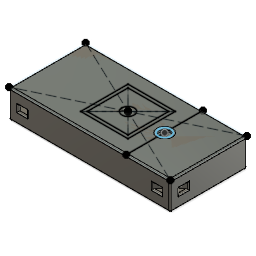
box1 (Autodesk Fusion 360 design; units mm, degrees)
Autodesk Fusion 360 part; units mm, degrees
note: some values were not read from the file. Set by a fixed rule: which sketch regions a step uses.
sketch "Sketch1" plane through (0, 0, 0) normal (0, 1, 0) x (1, 0, 0)
  line L0 (-95, -45) -> (95, -45)
  line L1 (95, -45) -> (95, 45)
  line L2 (95, 45) -> (-95, 45)
  line L3 (-95, 45) -> (-95, -45)
  line L4 (-95, -45) -> (95, 45) construction
  line L5 (95, -45) -> (-95, 45) construction
  line L6 (-99, -49) -> (99, -49)
  line L7 (99, -49) -> (99, 49)
  line L8 (99, 49) -> (-99, 49)
  line L9 (-99, 49) -> (-99, -49)
  line L10 (-99, -49) -> (99, 49) construction
  line L11 (99, -49) -> (-99, 49) construction
  line L12 (-57.3192, 45) -> (-19.6385, 45)
  line L13 (-19.6385, 45) -> (-19.6385, -45)
  line L14 (-19.6385, -45) -> (-57.3192, -45)
  line L15 (-57.3192, -45) -> (-57.3192, 45)
  line L16 (19.6385, 45) -> (57.3192, 45)
  line L17 (57.3192, 45) -> (57.3192, -45)
  line L18 (57.3192, -45) -> (19.6385, -45)
  line L19 (19.6385, -45) -> (19.6385, 45)
  line L20 (-57.3192, -35) -> (-19.6385, -35) construction
  line L21 (19.6385, -35) -> (57.3192, -35) construction
  line L22 (57.3192, -20) -> (95, -20) construction
  line L23 (-95, -29.9905) -> (-57.3192, -29.9905) construction
  line L24 (-87.5, 49) -> (87.5, 49)
  line L25 (-99, -49) -> (99, -49)
  line L26 (99, -49) -> (99, -143)
  line L27 (99, -143) -> (-99, -143)
  line L28 (-99, -143) -> (-99, -49)
  line L29 (-95, -49) -> (95, -49)
  line L30 (95, -49) -> (95, -139)
  line L31 (95, -139) -> (-95, -139)
  line L32 (-95, -139) -> (-95, -49)
  line L33 (-95, -49) -> (-75, -49)
  line L34 (-75, -49) -> (-75, -74)
  line L35 (-75, -74) -> (-95, -74)
  line L36 (-95, -74) -> (-95, -49)
  line L37 (-95, -139) -> (-75, -139)
  line L38 (-75, -139) -> (-75, -119)
  line L39 (-75, -119) -> (-95, -119)
  line L40 (-95, -119) -> (-95, -139)
  line L41 (95, -139) -> (75, -139)
  line L42 (75, -139) -> (75, -119)
  line L43 (75, -119) -> (95, -119)
  line L44 (95, -119) -> (95, -139)
  line L45 (95, -49) -> (75, -49)
  line L46 (75, -49) -> (75, -74)
  line L47 (75, -74) -> (95, -74)
  line L48 (95, -74) -> (95, -49)
  dimension "d1" = 190
  dimension "d2" = 90
  dimension "d4" = 4
  dimension "d5" = 4
  dimension "d26" = 4
  dimension "d27" = 4
  dimension "d28" = 4
  dimension "d29" = 20
  dimension "d30" = 25
  dimension "d31" = 20
  dimension "d32" = 20
  dimension "d33" = 20
  dimension "d34" = 20
  dimension "d35" = 20
  dimension "d36" = 25
  dimension "d48" = 90
  constraint horizontal L0
  constraint perpendicular L0 L1
  constraint parallel L0 L2
  constraint parallel L1 L3
  constraint coincident L4 origin
  constraint coincident L5 origin
  constraint horizontal L6
  constraint perpendicular L6 L7
  constraint parallel L6 L8
  constraint parallel L7 L9
  constraint coincident L10 origin
  constraint coincident L11 origin
  constraint horizontal L12
  constraint vertical L13
  constraint horizontal L14
  constraint vertical L15
  constraint coincident L0 L13.end
  constraint coincident L2 L12.start
  constraint horizontal L16
  constraint vertical L17
  constraint horizontal L18
  constraint vertical L19
  constraint coincident L0 L17.end
  constraint coincident L2 L16.start
  constraint coincident L13 L20.end
  constraint perpendicular L13 L20
  constraint coincident L19 L21.start
  constraint coincident L17 L21.end
  constraint perpendicular L17 L21
  constraint coincident L17 L22.start
  constraint coincident L1 L22.end
  constraint perpendicular L1 L22
  constraint coincident L15 L20.start
  constraint equal L20 L21
  constraint equal L21 L22
  constraint coincident L3 L23.start
  constraint coincident L15 L23.end
  constraint perpendicular L15 L23
  constraint equal L20 L23
  constraint horizontal L24
  constraint coincident L8 L24.start
  constraint horizontal L25
  constraint vertical L26
  constraint horizontal L27
  constraint vertical L28
  constraint collinear L7 L26
  constraint horizontal L29
  constraint vertical L30
  constraint horizontal L31
  constraint vertical L32
  constraint coincident L6 L29.start
  constraint horizontal L33
  constraint vertical L34
  constraint horizontal L35
  constraint vertical L36
  constraint horizontal L37
  constraint vertical L38
  constraint horizontal L39
  constraint vertical L40
  constraint horizontal L41
  constraint vertical L42
  constraint horizontal L43
  constraint vertical L44
  constraint horizontal L45
  constraint vertical L46
  constraint horizontal L47
  constraint vertical L48
  measures "d1" distance of L1.end L2.end
  measures "d2" distance of L0.end L1.end
  measures "d4" distance of L2 L8
  measures "d5" distance of L3 L9
  measures "d26" distance of L26 L30
  measures "d27" distance of L28 L32
  measures "d28" distance of L27 L31
  measures "d29" distance of L29.start L33.end
  measures "d30" distance of L29.start L35.end
  measures "d31" distance of L31.end L37.end
  measures "d32" distance of L31.end L39.end
  measures "d33" distance of L30.end L41.end
  measures "d34" distance of L30.end L43.end
  measures "d35" distance of L29.end L45.end
  measures "d36" distance of L29.end L47.end
  measures "d48" distance of L25 L31
extrude "Extrude1" add sketch "Sketch1" along normal blind 31 from surface at 4 contours L6 L7 L8 L9 L24 L25 L29 L33 L45 makes body 1
extrude "Extrude2" add sketch "Sketch1" along normal blind 4 contours L0 L2 L3 L15 | L0 L2 L12 L13 L14 L15 | L0 L2 L13 L19 | L0 L2 L16 L17 L18 L19 | L0 L1 L2 L17 | L6 L7 L8 L9 L24 L25 L29 L33 L45 bodies 1
sketch "Sketch2" plane through (-99, 0, 0) normal (-1, 0, 0) x (0, 0, 1)
  line L0 (49, 0) -> (49, 35)
  line L1 (49, 35) -> (-49, 35)
  line L2 (-49, 35) -> (-49, 0)
  line L3 (-49, 0) -> (49, 0)
  line L4 (-45, 4) -> (45, 4)
  line L5 (45, 4) -> (45, 31)
  line L6 (45, 31) -> (-45, 31)
  line L7 (-45, 31) -> (-45, 4)
  line L8 (-45, 4) -> (45, 31) construction
  line L9 (45, 4) -> (-45, 31) construction
  line L10 (-49, 35) -> (49, 0) construction
  line L11 (-49, 0) -> (49, 35) construction
  line L12 (-49, 0) -> (49, 0)
  point P0 (0, 17.5)
  point P1 (0, 17.5)
  dimension "d12" = 90
  dimension "d15" = 4
  constraint horizontal L4
  constraint perpendicular L4 L5
  constraint parallel L4 L6
  constraint parallel L5 L7
  constraint coincident L8 P1
  constraint coincident L9 P1
  constraint coincident L1.end L2.start
  constraint coincident L0.start L3.end
  constraint coincident L2.end L3.start
  constraint coincident L0.end L1.start
  constraint midpoint L10 P1
  constraint coincident P1 P0
  measures "d12" distance of L5 L7
  measures "d15" distance of L4 L12
extrude "Extrude3" cut sketch "Sketch2" against normal blind 10 contours L4 L5 L6 L7 bodies 1
sketch "Sketch3" plane through (0, 0, 0) normal (0, 1, 0) x (1, 0, 0)
extrude "Extrude4" cut sketch "Sketch1" along normal blind 20 contours L0 L2 L3 L15 | L0 L2 L13 L19 | L0 L1 L2 L17 bodies 1
sketch "Sketch5" plane through (0, 0, -49) normal (0, 0, -1) x (-1, 0, 0)
  line L0 (99, 0) -> (99, 35)
  line L1 (99, 35) -> (-99, 35)
  line L2 (-99, 35) -> (-99, 0)
  line L3 (-99, 0) -> (99, 0)
  line L4 (-79, 15) -> (99, 15)
  line L5 (99, 15) -> (99, 20)
  line L6 (99, 20) -> (-79, 20)
  line L7 (-79, 20) -> (-79, 15)
  line L8 (-79, 15) -> (99, 20) construction
  line L9 (99, 15) -> (-79, 20) construction
  line L10 (-9.2061, 20) -> (-9.2061, 35) construction
  line L11 (-3.2436, 15) -> (-3.2436, 0) construction
  point P0 (0, 17.5)
  point P1 (10, 17.5)
  dimension "d18" = 5
  dimension "d22" = 20
  constraint horizontal L4
  constraint perpendicular L4 L5
  constraint parallel L4 L6
  constraint parallel L5 L7
  constraint coincident L8 P1
  constraint coincident L9 P1
  constraint collinear L0 L5
  constraint coincident L6 L10.start
  constraint coincident L1 L10.end
  constraint perpendicular L1 L10
  constraint coincident L4 L11.start
  constraint coincident L3 L11.end
  constraint perpendicular L3 L11
  constraint equal L10 L11
  measures "d18" distance of L4.end L5.end
  measures "d22" distance of L2 L7
extrude "Extrude5" cut sketch "Sketch5" against normal blind 25 contours L0 L4 L5 L6 L7 bodies 1
extrude "Extrude7" add sketch "Sketch1" along normal blind 4 contours L6 L25 L26 L27 L28 L30 L31 L32 L36 L37 L40 L41 L44 L48 | L6 L25 L29 L32 L33 L34 L35 L36 | L6 L25 L29 L30 L31 L32 L34 L35 L38 L39 L42 L43 L46 L47 | L6 L25 L29 L30 L45 L46 L47 L48 | L31 L32 L37 L38 L39 L40 | L30 L31 L41 L42 L43 L44 bodies 1
extrude "Extrude8" add sketch "Sketch1" along normal blind 27 from surface at 4 contours L6 L25 L26 L27 L28 L30 L31 L32 L36 L37 L40 L41 L44 L48 | L6 L25 L29 L32 L33 L34 L35 L36 | L6 L25 L29 L30 L45 L46 L47 L48 | L31 L32 L37 L38 L39 L40 | L30 L31 L41 L42 L43 L44 bodies 1
extrude "Extrude9" add sketch "Sketch1" along normal blind 4 from surface at 31 contours L6 L25 L26 L27 L28 L30 L31 L32 L36 L37 L40 L41 L44 L48 | L6 L25 L29 L32 L33 L34 L35 L36 | L6 L25 L29 L30 L31 L32 L34 L35 L38 L39 L42 L43 L46 L47 | L6 L25 L29 L30 L45 L46 L47 L48 | L31 L32 L37 L38 L39 L40 | L30 L31 L41 L42 L43 L44 bodies 1
ref_plane "WorkPlane1" through (-2, 17.5, 49) normal (0, 0, -1) x (-1, 0, 0)
split "Split1" by plane through (-2, 17.5, 49) normal (0, 0, -1) bodies 1 makes body 2 at (-32.1987, 0, 15)
sketch "Sketch6" plane through (-2, 17.5, 49) normal (0, 0, -1) x (1, 0, 0)
  line L0 (84.4427, 6.7781) -> (87.2066, 6.5756)
  line L1 (87.2066, 6.5756) -> (88.7639, 8.8679)
  line L2 (88.7639, 8.8679) -> (87.5574, 11.3627)
  line L3 (87.5574, 11.3627) -> (84.7936, 11.5653)
  line L4 (84.7936, 11.5653) -> (83.2362, 9.273)
  line L5 (83.2362, 9.273) -> (84.4427, 6.7781)
  line L6 (86.9405, -6.4213) -> (84.2127, -6.9103)
  line L7 (84.2127, -6.9103) -> (83.2723, -9.5172)
  line L8 (83.2723, -9.5172) -> (85.0597, -11.635)
  line L9 (85.0597, -11.635) -> (87.7875, -11.146)
  line L10 (87.7875, -11.146) -> (88.7279, -8.5391)
  line L11 (88.7279, -8.5391) -> (86.9405, -6.4213)
  line L12 (-80.9611, -6.4547) -> (-83.7039, -6.8509)
  line L13 (-83.7039, -6.8509) -> (-84.7323, -9.4243)
  line L14 (-84.7323, -9.4243) -> (-83.0178, -11.6016)
  line L15 (-83.0178, -11.6016) -> (-80.275, -11.2054)
  line L16 (-80.275, -11.2054) -> (-79.2466, -8.632)
  line L17 (-79.2466, -8.632) -> (-80.9611, -6.4547)
  line L18 (-80.9482, 11.6387) -> (-83.693, 11.2563)
  line L19 (-83.693, 11.2563) -> (-84.7342, 8.6881)
  line L20 (-84.7342, 8.6881) -> (-83.0307, 6.5022)
  line L21 (-83.0307, 6.5022) -> (-80.2859, 6.8846)
  line L22 (-80.2859, 6.8846) -> (-79.2447, 9.4528)
  line L23 (-79.2447, 9.4528) -> (-80.9482, 11.6387)
  line L24 (-81.9895, 9.0704) -> (-81.9895, -9.0282) construction
  line L25 (86.0001, 9.0704) -> (86.0001, -9.0282) construction
  line L26 (86.0001, -9.0282) -> (-81.9895, -9.0282) construction
  line L27 (-81.9895, 9.0704) -> (86.0001, 9.0704) construction
  circle A0 centre (86.0001, -9.0282) radius 1.75
  circle A1 centre (86.0001, 9.0704) radius 1.75
  circle A2 centre (-81.9895, 9.0704) radius 1.75
  circle A3 centre (-81.9895, -9.0282) radius 1.75
  circle A4 centre (-81.9895, -9.0282) radius 3.5
  circle A5 centre (-81.9895, 9.0704) radius 3.5
  circle A6 centre (86.0001, -9.0282) radius 3.5
  circle A7 centre (86.0001, 9.0704) radius 3.5
  point P0 (86.0001, 9.0704)
  point P1 (86.0001, -9.0282)
  point P2 (-81.9895, -9.0282)
  point P3 (-81.9895, 9.0704)
  dimension "d49" = 4.8
  dimension "d50" = 4.8
  dimension "d51" = 4.8
  dimension "d52" = 4.8
  dimension "d55" = 3.5
  dimension "d56" = 3.5
  dimension "d57" = 3.5
  dimension "d58" = 3.5
  dimension "d63" = 7
  dimension "d64" = 7
  dimension "d65" = 7
  dimension "d66" = 7
  constraint coincident P3 L24.start
  constraint coincident P2 L24.end
  constraint vertical L24
  constraint coincident P0 L25.start
  constraint coincident P1 L25.end
  constraint vertical L25
  constraint horizontal L27
  constraint horizontal L26
  measures "d49" distance of L0 L3
  measures "d50" distance of L8 L11
  measures "d51" distance of L13 L16
  measures "d52" distance of L20 L23
  measures "d55" diameter of A0
  measures "d56" diameter of A1
  measures "d57" diameter of A2
  measures "d58" diameter of A3
  measures "d63" diameter of A4
  measures "d64" diameter of A5
  measures "d65" diameter of A6
  measures "d66" diameter of A7
extrude "Extrude10" cut sketch "Sketch6" against normal blind 3.5 contours L0 L1 L2 L3 L4 L5 | L6 L7 L8 L9 L10 L11 | L12 L13 L14 L15 L16 L17 | L18 L19 L20 L21 L22 L23 | A0 | A1 | A2 | A3 bodies 1
extrude "Extrude11" cut sketch "Sketch6" against normal blind 37 contours A0 | A1 | A2 | A3 bodies 1
extrude "Extrude12" cut sketch "Sketch6" along normal blind 1 contours A0 | A1 | A2 | A3 bodies 2
extrude "Extrude13" cut sketch "Sketch6" along normal blind 10 from surface at 1 contours L0 L1 L2 L3 L4 L5 | L6 L7 L8 L9 L10 L11 | L12 L13 L14 L15 L16 L17 | L18 L19 L20 L21 L22 L23 | A0 | A1 | A2 | A3 | A4 | A5 | A6 | A7 bodies 2
sketch "Sketch7" plane through (0, 35, 0) normal (0, 1, 0) x (-1, 0, 0)
  line L0 (-99, 49) -> (99, 49)
  line L1 (99, 49) -> (99, 143)
  line L2 (99, 143) -> (-99, 143)
  line L3 (-99, 143) -> (-99, 49)
  line L4 (99, 49) -> (-99, 143) construction
  line L5 (-99, 49) -> (99, 143) construction
  circle A0 centre (0, 96) radius 7.5
  line L6 (25, 121) -> (-25, 121)
  line L7 (-25, 121) -> (-25, 71)
  line L8 (-25, 71) -> (25, 71)
  line L9 (25, 71) -> (25, 121)
  line L10 (25, 121) -> (-25, 71) construction
  line L11 (-25, 121) -> (25, 71) construction
  line L12 (29, 125) -> (-29, 125)
  line L13 (-29, 125) -> (-29, 67)
  line L14 (-29, 67) -> (29, 67)
  line L15 (29, 67) -> (29, 125)
  line L16 (29, 125) -> (-29, 67) construction
  line L17 (-29, 125) -> (29, 67) construction
  circle A1 centre (-45, 96) radius 7.5
  line L18 (-45, 96) -> (-45, 49)
  line L19 (-45, 96) -> (-45, 143)
  point P0 (0, 96)
  point P1 (0, 96)
  point P2 (0, 96)
  dimension "d70" = 15
  dimension "d78" = 50
  dimension "d79" = 50
  dimension "d101" = 4
  dimension "d102" = 4
  dimension "d103" = 15
  dimension "d104" = 54
  constraint coincident L0.end L1.start
  constraint coincident L2.end L3.start
  constraint coincident L0.start L3.end
  constraint coincident L1.end L2.start
  constraint midpoint L4 P2
  constraint coincident P2 P1
  constraint horizontal L6
  constraint perpendicular L6 L7
  constraint parallel L6 L8
  constraint parallel L7 L9
  constraint coincident L10 P2
  constraint coincident L11 P2
  constraint horizontal L12
  constraint perpendicular L12 L13
  constraint parallel L12 L14
  constraint parallel L13 L15
  constraint coincident L16 P2
  constraint coincident L17 P2
  constraint coincident A1.centre L18.start
  constraint coincident L0 L18.end
  constraint coincident L2 L19.end
  constraint parallel L3 L19
  constraint parallel L3 L18
  constraint equal L18 L19
  measures "d70" diameter of A0
  measures "d78" distance of L7.end L8.end
  measures "d79" distance of L6.end L7.end
  measures "d101" distance of L9 L15
  measures "d102" distance of L8 L14
  measures "d103" diameter of A1
  measures "d104" distance of L3 A1.centre
sketch "Sketch8" plane through (0, 0, 45) normal (0, 0, -1) x (-1, 0, 0)
  circle A0 centre (-84.0001, 26.5282) radius 3.5
  circle A1 centre (83.9895, 26.5282) radius 3.5
  circle A2 centre (-84.0001, 8.4296) radius 3.5
  circle A3 centre (83.9895, 8.4296) radius 3.5
  line L0 (95, 4) -> (99, 4)
  line L1 (99, 4) -> (99, 31)
  line L2 (99, 31) -> (95, 31)
  line L3 (95, 31) -> (95, 35)
  line L4 (95, 35) -> (-95, 35)
  line L5 (-95, 35) -> (-95, 0)
  line L6 (-95, 0) -> (-57.3192, 0)
  line L7 (-57.3192, 0) -> (-57.3192, 4)
  line L8 (-57.3192, 4) -> (-19.6385, 4)
  line L9 (-19.6385, 4) -> (-19.6385, 0)
  line L10 (-19.6385, 0) -> (19.6385, 0)
  line L11 (19.6385, 0) -> (19.6385, 4)
  line L12 (19.6385, 4) -> (57.3192, 4)
  line L13 (57.3192, 4) -> (57.3192, 0)
  line L14 (57.3192, 0) -> (95, 0)
  line L15 (95, 0) -> (95, 4)
  line L16 (50.1642, 12.9509) -> (70.1642, 12.9509)
  line L17 (70.1642, 12.9509) -> (70.1642, 22.9509)
  line L18 (70.1642, 22.9509) -> (50.1642, 22.9509)
  line L19 (50.1642, 22.9509) -> (50.1642, 12.9509)
  dimension "d73" = 20
  dimension "d74" = 10
  constraint horizontal L16
  constraint vertical L17
  constraint horizontal L18
  constraint vertical L19
  measures "d73" distance of L16.start L16.end
  measures "d74" distance of L16.start L18.end
extrude "Extrude15" cut sketch "Sketch8" against normal blind 10 contours L16 L17 L18 L19 bodies 2
sketch "Sketch9" plane through (0, 35, 0) normal (0, 1, 0) x (-1, 0, 0)
  line L0 (-99, 49) -> (99, 49)
  line L1 (99, 49) -> (99, 143)
  line L2 (99, 143) -> (-99, 143)
  line L3 (-99, 143) -> (-99, 49)
  line L4 (73.6899, 145.6827) -> (104.7545, 114.6181)
  line L5 (108.9838, 118.8741) -> (79.3624, 148.4954)
  line L6 (108.9838, 118.8741) -> (104.7545, 114.6181)
  line L7 (79.3624, 148.4954) -> (73.6899, 145.6827)
  line L8 (-102.3752, 116.9974) -> (-70.3563, 149.0163)
  line L9 (-76.0637, 151.7942) -> (-105.7736, 122.0843)
  line L10 (-99, 143) -> (99, 143)
  line L11 (-99, 49) -> (-99, 143)
  line L12 (-105.7736, 122.0843) -> (-102.3752, 116.9974)
  line L13 (-76.0637, 151.7942) -> (-70.3563, 149.0163)
  dimension "d86" = 6
  dimension "d87" = 10
  dimension "d88" = 6
  dimension "d89" = 10
  dimension "d90" = 45
  dimension "d91" = 45
  constraint parallel L4 L5
  constraint parallel L8 L9
  measures "d86" distance of L4 L5
  measures "d87" distance of L1.end L5
  measures "d88" distance of L8 L9
  measures "d89" distance of L2.end L9
  measures "d90" angle of L5 L10
  measures "d91" angle of L9 L11
extrude "Extrude17" cut sketch "Sketch9" against normal blind 6 from surface at -14.5 contours L3 L8 L9 L11 L12 | L2 L3 L8 L9 L10 L11 | L1 L2 L4 L5 L10 | L1 L4 L5 L6 | L2 L8 L9 L10 L13 | L2 L4 L5 L7 L10 bodies 1
extrude "Extrude19" cut sketch "Sketch7" against normal blind 6 contours A1 L18 L19 | A1 L18 L19 bodies 1
fillet "Fillet3" radius 2 5 faces at (99, 16.5, 72.7909) (-53.5, 35, 96) (25.4575, 30.1667, 143) (-99, 16.5, 72.7909) (33, 0, 111.6667) on bodies 1
hidden bodies 2
equation "e = 4 mm"
equation "d4 = e"
equation "d5 = e"
equation "d6 = e"
equation "d7 = 27 mm + e"
equation "d9 = e"
equation "d15 = e"
equation "d26 = e"
equation "d27 = e"
equation "d28 = e"
equation "d39 = e"
equation "d41 = e"
equation "d44 = e + 27 mm"
equation "d45 = e"
equation "d47 = -e"
equation "d101 = e"
equation "d102 = e"
equation "d104 = e + 50 mm"
named bodies: "BoitePhoto", "BoiteBatterie"
